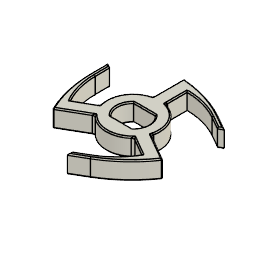
Pawl (Autodesk Fusion 360 design; units mm, degrees)
Autodesk Fusion 360 part; units mm, degrees
sketch "Spring_Pawl_Sketch" plane through (0, 0, 0) normal (0, 0, 1) x (1, 0, 0)
  line L0 (-3.0817, 3.2) -> (3.0817, 3.2)
  arc A0 (-3.0817, 3.2) -> (-3.0817, -3.2) centre (0, 0) ccw
  arc A1 (3.0817, -3.2) -> (3.0817, 3.2) centre (0, 0) ccw
  line L1 (3.0817, -3.2) -> (-3.0817, -3.2)
  circle A2 centre (0, 0) radius 7.5
  line L2 (16.0522, 9.4987) -> (14.8475, 8.8032)
  line L3 (11.922, 11.847) -> (16.0522, 9.4987)
  line L4 (11.3289, 10.8038) -> (14.8475, 8.8032)
  line L5 (1.75, 7.293) -> (1.75, 13.3861)
  line L6 (-1.75, 7.293) -> (-1.75, 16)
  arc A3 (11.922, 11.847) -> (-1.75, 16) centre (-4.1103, -16.3509) ccw
  arc A4 (11.3289, 10.8038) -> (1.75, 13.3861) centre (1.5589, -6.3798) ccw
  line L7 (-7.1909, -2.1309) -> (-12.4677, -5.1775)
  line L8 (-5.4409, -5.162) -> (-12.9814, -9.5155)
  arc A5 (-16.2207, 4.4012) -> (-12.9814, -9.5155) centre (16.2155, 4.6159) ccw
  arc A6 (-15.0208, 4.4092) -> (-12.4677, -5.1775) centre (4.7457, 4.54) ccw
  line L9 (-15.0208, 4.4092) -> (-15.0475, 8.4568)
  line L10 (-16.2207, 4.4012) -> (-16.2522, 9.1523)
  line L11 (-16.2522, 9.1523) -> (-15.0475, 8.4568)
  line L12 (5.4409, -5.162) -> (10.7177, -8.2086)
  line L13 (7.1909, -2.1309) -> (14.7314, -6.4845)
  arc A7 (4.2988, -16.2482) -> (14.7314, -6.4845) centre (-12.1052, 11.7351) ccw
  arc A8 (3.6919, -15.213) -> (10.7177, -8.2086) centre (-6.3046, 1.8399) ccw
  line L14 (3.6919, -15.213) -> (0.2, -17.2599)
  line L15 (4.2988, -16.2482) -> (0.2, -18.6509)
  line L16 (0.2, -18.6509) -> (0.2, -17.2599)
  dimension "d3" = 15
  dimension "d9" = 360
  constraint coincident A2 L6.start
  constraint coincident A2 L5.start
  constraint tangent L3 A3
  constraint tangent L4 A4
  measures "d3" diameter of A2
extrude "Extrude1" add sketch "Spring_Pawl_Sketch" along normal blind 5
fillet "Fillet1" radius 0.3 2 faces at (0.1843, -4.6265, 5) (0.1843, -4.6265, 0)
fillet "Fillet2" radius 0.8 18 edges at (-7.0715, -2.1782, 0.0758) (-7.1909, -2.1309, 2.5) (-7.0715, -2.1782, 4.9242) (-5.4221, -5.035, 0.0758) (-5.4409, -5.162, 2.5) (-5.4221, -5.035, 4.9242) (5.4221, -5.035, 0.0758) (5.4409, -5.162, 2.5) (5.4221, -5.035, 4.9242) (7.0715, -2.1782, 0.0758) (7.1909, -2.1309, 2.5) (7.0715, -2.1782, 4.9242) (1.6494, 7.2132, 0.0758) (1.75, 7.293, 2.5) (1.6494, 7.2132, 4.9242) (-1.6494, 7.2132, 0.0758) (-1.75, 7.293, 2.5) (-1.6494, 7.2132, 4.9242)
fillet "Fillet3" radius 0.2 9 edges at (-12.9349, -9.3647, 0.07) (-12.9814, -9.5155, 2.5) (-12.9349, -9.3647, 4.93) (14.5775, -6.5196, 0.07) (14.7314, -6.4845, 2.5) (14.5775, -6.5196, 4.93) (-1.6426, 15.8843, 0.07) (-1.75, 16, 2.5) (-1.6426, 15.8843, 4.93)
named bodies: "Spring_Pawl_Body"
